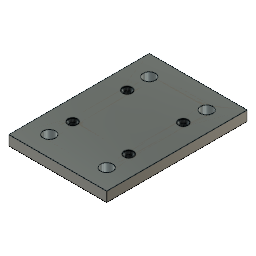
Y2023_P001_IMU_mount_v2 (Autodesk Fusion 360 design; units mm, degrees)
Autodesk Fusion 360 part; units mm, degrees
sketch "Sketch1" plane through (0, 0, 0) normal (0, 0, 1) x (1, 0, 0)
  line L0 (-34.15, 48.95) -> (34.15, 48.95)
  line L1 (34.15, 48.95) -> (34.15, -48.95)
  line L2 (34.15, -48.95) -> (-34.15, -48.95)
  line L3 (-34.15, -48.95) -> (-34.15, 48.95)
  line L4 (-34.15, 48.95) -> (34.15, -48.95) construction
  line L5 (34.15, 48.95) -> (-34.15, -48.95) construction
  line L6 (19.5, 19) -> (-19.5, 19) construction
  line L7 (-19.5, 19) -> (-19.5, -19) construction
  line L8 (-19.5, -19) -> (19.5, -19) construction
  line L9 (19.5, -19) -> (19.5, 19) construction
  line L10 (19.5, 19) -> (-19.5, -19) construction
  line L11 (-19.5, 19) -> (19.5, -19) construction
  circle A0 centre (-19.5, 19) radius 1.75
  circle A1 centre (19.5, 19) radius 1.75
  circle A2 centre (19.5, -19) radius 1.75
  circle A3 centre (-19.5, -19) radius 1.75
  line L12 (0, 1.75) -> (0, 22.5)
  line L13 (1.75, 0) -> (22.5, 0)
  line L14 (20, 34.8) -> (-20, 34.8) construction
  line L15 (-20, 34.8) -> (-20, -34.8) construction
  line L16 (-20, -34.8) -> (20, -34.8) construction
  line L17 (20, -34.8) -> (20, 34.8) construction
  line L18 (20, 34.8) -> (-20, -34.8) construction
  line L19 (-20, 34.8) -> (20, -34.8) construction
  circle A4 centre (-20, 34.8) radius 4.25
  circle A5 centre (20, 34.8) radius 4.25
  circle A6 centre (20, -34.8) radius 4.25
  circle A7 centre (-20, -34.8) radius 4.25
  dimension "d3" = 39
  dimension "d4" = 38
  dimension "d5" = 3.5
  dimension "d10" = 40
  dimension "d11" = 8.5
  dimension "d12" = 15.8
  dimension "d13" = 14.15
  dimension "d16" = 68.3
  constraint horizontal L0
  constraint perpendicular L0 L1
  constraint parallel L0 L2
  constraint parallel L1 L3
  constraint coincident L4 origin
  constraint coincident L5 origin
  constraint horizontal L6
  constraint perpendicular L6 L7
  constraint parallel L6 L8
  constraint parallel L7 L9
  constraint coincident L10 origin
  constraint coincident L11 origin
  constraint coincident L6.end L7.start
  constraint coincident L6.start L9.end
  constraint coincident L8.end L9.start
  constraint coincident L7.end L8.start
  constraint equal A0 A1
  constraint equal A2 A3
  constraint equal A0 A3
  constraint horizontal L14
  constraint perpendicular L14 L15
  constraint parallel L14 L16
  constraint parallel L15 L17
  constraint coincident L18 origin
  constraint coincident L19 origin
  constraint coincident L14.end L15.start
  constraint coincident L14.start L17.end
  constraint coincident L16.end L17.start
  constraint coincident L15.end L16.start
  constraint equal A4 A5
  constraint equal A5 A6
  constraint equal A6 A7
  measures "d3" distance of L6.start L6.end
  measures "d4" distance of L6.start L8.end
  measures "d5" diameter of A0
  measures "d10" distance of L14.start L14.end
  measures "d11" diameter of A4
  measures "d12" distance of L6 L14.end
  measures "d13" distance of L0 L14
  measures "d16" distance of L1 L3
extrude "Extrude2" add sketch "Sketch1" along normal blind 7
sketch "Sketch2" plane through (0, 0, 7) normal (0, 0, 1) x (-1, 0, 0)
  circle A0 centre (-19.5, 19) radius 1.75
  circle A1 centre (19.5, 19) radius 1.75
  circle A2 centre (19.5, -19) radius 1.75
  circle A3 centre (-19.5, -19) radius 1.75
  circle A4 centre (20, -34.8) radius 4.25
  circle A5 centre (-20, -34.8) radius 4.25
  circle A6 centre (-20, 34.8) radius 4.25
  circle A7 centre (20, 34.8) radius 4.25
  line L0 (34.15, 48.95) -> (-34.15, 48.95)
  line L1 (-34.15, 48.95) -> (-34.15, -48.95)
  line L2 (-34.15, -48.95) -> (34.15, -48.95)
  line L3 (34.15, -48.95) -> (34.15, 48.95)
  circle A8 centre (19.5, 19) radius 3
  circle A9 centre (-19.5, 19) radius 3
  circle A10 centre (-19.5, -19) radius 3
  circle A11 centre (19.5, -19) radius 3
  dimension "d17" = 6
  constraint concentric A1 A8
  constraint concentric A0 A9
  constraint concentric A3 A10
  constraint concentric A2 A11
  constraint equal A10 A11
  constraint equal A9 A10
  constraint equal A8 A9
  measures "d17" diameter of A11
hole "Hole1" at (19.5, 19, 7) direction (0, 0, -1) diameter 3 depth 10 tip angle 118 countersink diameter 6.5 countersink angle 90
hole "Hole2" at (-19.5, 19, 7) direction (0, 0, -1) diameter 3 depth 16 tip angle 118 countersink diameter 6.5 countersink angle 90
hole "Hole3" at (-19.5, -19, 7) direction (0, 0, -1) diameter 3 depth 16 tip angle 118 countersink diameter 6.5 countersink angle 90
hole "Hole4" at (19.5, -19, 7) direction (0, 0, -1) diameter 3 depth 16 tip angle 118 countersink diameter 6.5 countersink angle 90
equation "d12 = 10 mm + ( 3.3 / 2 ) * 1 mm + ( 8.3 / 2 ) * 1 mm"
equation "d13 = 10 mm + ( 8.3 / 2 ) * 1 mm"
equation "d16 = 40 mm + 8.3 mm + 20 mm"
